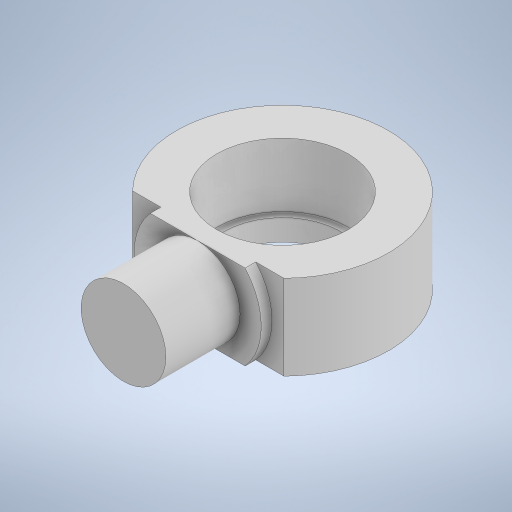
# Autodesk Inventor part: borde libre chico
Saved by Autodesk Inventor 2024 (Build 280153000, 153)
## iProperties
Created: 2024-04-11
Part Number: borde libre chico
Material: Generic
Document SubType Name: Modeling
Designer: compu
Density: 1 g/cm^3
Appearance: Default
Author: compu
Autodesk Inventor part; units mm, degrees
ref_plane "YZ Plane" through (0, 0, 0) normal (1, 0, 0) x (0, 1, 0)
ref_plane "XZ Plane" through (0, 0, 0) normal (0, 1, 0) x (-1, 0, 0)
ref_plane "XY Plane" through (0, 0, 0) normal (0, 0, 1) x (1, 0, 0)
sketch "Sketch1" plane through (0, 0, 0) normal (0, 1, 0) x (-1, 0, 0)
  line L0 (0, -19.6) -> (0, 19.6) projected
  line L1 (19.6, 0) -> (-19.6, 0) projected
  circle A0 centre (0, 0) radius 2
  circle A1 centre (0, 0) radius 6.2
  circle A2 centre (0, 0) radius 14
  line L2 (4, -13.4164) -> (-4, -13.4164)
  circle A3 centre (0, 0) radius 10
  line L3 (6, 8) -> (-6, 8)
  line L4 (7.1414, 7) -> (-7.1414, 7)
  dimension "d0" = 4
  dimension "d1" = 12.4
  dimension "d2" = 28
  dimension "d3" = 8
  dimension "d4" = 20
  dimension "d5" = 12
  dimension "d7" = 1
  constraints: 6 end point, 6 point on circle, 4 centre point, 4 coincident, 3 horizontal, 1 perpendicular
  measures "d0" diameter of A0
  measures "d1" diameter of A1
  measures "d2" diameter of A2
  measures "d3" distance of L2.start L2.end
  measures "d4" diameter of A3
  measures "d5" distance of L3.start L3.end
  measures "d7" distance between parallel lines of L3 L4
extrude "Extrusion1" add sketch "Sketch1" along normal blind 8 contours A3 L1 A1 L0 | L0 A1 L1 A3 | A3 L4 L0 A1 L1 | L1 A1 L0 L4 A3
sketch "Sketch2" plane through (-7.1414, 0, 7) normal (0, 0, 1) x (1, 0, 0)
  line L0 (0, 0) -> (14.2829, 0) projected
  line L1 (14.2829, 0) -> (14.2829, 8) projected
  line L2 (0, 8) -> (14.2829, 8) projected
  line L3 (0, 0) -> (0, 8) projected
  line L4 (7.1414, -4) -> (7.1414, 10) projected
  line L5 (2.6693, 8) -> (11.6136, 8)
  line L6 (2.6693, 0) -> (11.6136, 0)
  arc A0 (2.6693, 8) -> (2.6693, 0) centre (7.1414, 4) ccw
  arc A1 (11.6136, 0) -> (11.6136, 8) centre (7.1414, 4) ccw
  point P0 (7.1414, 0)
  dimension "d10" = 4
  dimension "d26" = 8
  dimension "d27" = 6
  dimension "d28" = 6
  constraints: 4 end point, 4 point on circle, 2 centre point, 2 horizontal, 1 coincident, 1 parallel, 1 point on line
  measures "d10" distance from line of L0 point (7.141, 4)
  measures "d26" distance between parallel lines of L6 L5
  measures "d27" radius of A1
  measures "d28" radius of A0
extrude "Extrusion2" add sketch "Sketch2" along normal blind 1 contours A0 L2 L4 L0 | L4 L2 A1 L0
sketch "Sketch3" plane through (-7.1414, 0, 8) normal (0, 0, 1) x (1, 0, 0)
  arc A0 (2.6693, 8) -> (2.6693, 0) centre (7.1414, 4) ccw projected
  circle A1 centre (7.1414, 4) radius 4
  point P0 (7.1414, 0)
  point P1 (6.5905, 0)
  point P2 (6.5905, 4)
  dimension "d14" = 8
  constraints: 2 coincident, 1 centre point, 1 other
  measures "d14" diameter of A1
extrude "Extrusion3" add sketch "Sketch3" along normal blind 7
sketch "Sketch4" plane through (0, 0, 0) normal (0, 1, 0) x (-1, 0, 0)
  circle A0 centre (0, 0) radius 5.5
  circle A1 centre (0, 0) radius 6.2 projected
  circle A2 centre (0, 0) radius 6.5
  dimension "d29" = 11
  dimension "d30" = 13
  constraints: 2 centre point, 2 concentric
  measures "d29" diameter of A0
  measures "d30" diameter of A2
extrude "Extrusion4" add sketch "Sketch4" along normal blind 2 contours A1
body "Solid1"
